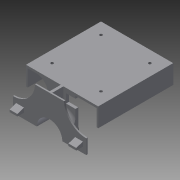
# Autodesk Inventor part: irkit-holder
Saved by Autodesk Inventor 2014 SP2 (Build 180247200, 247)
## iProperties
Created: 2017-11-24
Part Number: irkit-holder
Material: 一般
Document SubType Name: Modeling
Designer: hide
Density: 1 g/cm^3
Appearance: 既定
Author: hide
Autodesk Inventor part; units mm, degrees
ref_plane "YZ Plane" through (0, 0, 0) normal (1, 0, 0) x (0, 1, 0)
ref_plane "XZ Plane" through (0, 0, 0) normal (0, 1, 0) x (-1, 0, 0)
ref_plane "XY Plane" through (0, 0, 0) normal (0, 0, 1) x (1, 0, 0)
sketch "スケッチ1" plane through (0, 0, 0) normal (0, 1, 0) x (-1, 0, 0)
  arc A0 (11.5, 0) -> (-11.5, 0) centre (0, 0) ccw
  arc A1 (13, 0) -> (-13, 0) centre (0, 0) ccw
  line L0 (-13, 0) -> (-11.5, 0)
  line L1 (11.5, 0) -> (13, 0)
  dimension "d0" = 1.5
  dimension "d1" = 23
  constraints: 4 end point, 4 point on circle, 2 centre point, 2 coincident, 2 horizontal
  measures "d0" radial gap between concentric circles of A0 A1
  measures "d1" diameter of A0
extrude "押し出し1" add sketch "スケッチ1" along normal blind 12.5
sketch "スケッチ2" plane through (0, 12.5, 0) normal (0, 1, 0) x (1, 0, 0)
  arc A0 (-13, 0) -> (13, 0) centre (0, 0) ccw projected
  line L0 (13, 0) -> (11.5, 0) projected
  arc A1 (-11.5, 0) -> (11.5, 0) centre (0, 0) ccw projected
  line L1 (-11.5, 0) -> (-13, 0) projected
  line L2 (12, 0) -> (12, -30)
  line L3 (12, -30) -> (-13, -30)
  line L4 (-13, -30) -> (-13, 0)
  line L5 (-13, 0) -> (-11.5, 0)
  line L6 (11.5, 0) -> (12, 0)
  line L7 (12, -19.8001) -> (3.5501, -19.8001)
  line L8 (3.5501, -19.8001) -> (3.5501, -27.7778)
  line L9 (3.5501, -27.7778) -> (12, -27.7778)
  line L10 (12, -27.7778) -> (12, -19.8001)
  dimension "d4" = 30
  constraints: 18 end point, 5 parallel, 3 horizontal, 3 perpendicular, 2 point on circle, 1 point on line
  measures "d4" distance of L3.end L1.end
extrude "押し出し2" add sketch "スケッチ2" against normal blind 2.5 contours A0 L2 L7 L8 L9 L3 L4
sketch "スケッチ3" plane through (-13, 12.5, 30) normal (0, 0, 1) x (1, 0, 0)
  line L0 (0, 0) -> (25, 0) projected
  line L1 (25, -2.5) -> (0, -2.5) projected
  line L2 (-19.5, -2.5) -> (45.5, -2.5)
  line L3 (45.5, -2.5) -> (45.5, 65)
  line L4 (45.5, 65) -> (-19.5, 65)
  line L5 (-19.5, 65) -> (-19.5, -2.5)
  circle A0 centre (-9, 54.5) radius 1.25
  circle A1 centre (35, 54.5) radius 1.25
  circle A2 centre (-9, 10.5) radius 1.25
  circle A3 centre (35, 10.5) radius 1.25
  point P0 (13, -12.5)
  dimension "d7" = 65
  dimension "d8" = 0
  dimension "d9" = 65
  dimension "d10" = 32.5
  dimension "d13" = 2.5
  dimension "d14" = 2.5
  dimension "d15" = 2.5
  dimension "d16" = 2.5
  dimension "d17" = 44
  dimension "d18" = 44
  dimension "d19" = 0
  dimension "d20" = 0
  dimension "d21" = 10.5
  dimension "d22" = 10.5
  dimension "d23" = 44
  dimension "d24" = 0
  constraints: 8 end point, 4 centre point, 2 parallel, 1 horizontal, 1 perpendicular
  measures "d7" distance of L3.end L4.end
  measures "d8" distance between parallel lines of L1 L2
  measures "d9" distance between parallel lines of L0 L4
  measures "d10" distance from line of point (13, -12.5) L5
  measures "d13" diameter of A0
  measures "d14" diameter of A1
  measures "d15" diameter of A2
  measures "d16" diameter of A3
  measures "d17" distance of A1.centre A0.centre
  measures "d18" distance of A3.centre A1.centre
  measures "d19" vertical distance of A3.centre A2.centre
  measures "d20" vertical distance of A1.centre A0.centre
  measures "d21" distance from line of L4 A0.centre
  measures "d22" distance from line of L5 A0.centre
  measures "d23" distance of A2.centre A3.centre
  measures "d24" horizontal distance of A0.centre A2.centre
extrude "押し出し3" add sketch "スケッチ3" along normal blind 2
fillet "フィレット1" radius 10 1 edges at (-13, 11.25, 30)
sketch "スケッチ5" plane through (-13, 12.5, 30) normal (0, 0, -1) x (-1, 0, 0)
  line L0 (19.5, -2.5) -> (10, -2.5) projected
  line L1 (19.5, 65) -> (19.5, -2.5) projected
  line L2 (-25, -2.5) -> (-45.5, -2.5) projected
  line L3 (-45.5, 65) -> (-44, 65)
  line L4 (-44, 65) -> (-44, -2.5)
  line L5 (-44, -2.5) -> (-45.5, -2.5)
  line L6 (-45.5, -2.5) -> (-45.5, 65)
  line L7 (19.5, 65) -> (18, 65)
  line L8 (18, 65) -> (18, -2.5)
  line L9 (18, -2.5) -> (19.5, -2.5)
  line L10 (19.5, -2.5) -> (19.5, 65)
  point P0 (-13, -12.5)
  dimension "d26" = 1.5
  dimension "d27" = 1.5
  constraints: 16 end point, 4 parallel, 2 horizontal, 2 perpendicular, 2 point on line
  measures "d26" distance between parallel lines of L6 L4
  measures "d27" distance between parallel lines of L1 L8
extrude "押し出し4" add sketch "スケッチ5" along normal blind 15
sketch "スケッチ6" plane through (-13, 12.5, 30) normal (0, 0, -1) x (-1, 0, 0)
  circle A0 centre (-35, 10.5) radius 1.25 projected
  circle A1 centre (9, 10.5) radius 1.25 projected
  circle A2 centre (-35, 54.5) radius 1.25 projected
  circle A3 centre (9, 54.5) radius 1.25 projected
  circle A4 centre (-35, 54.5) radius 2.5
  circle A5 centre (-35, 10.5) radius 2.5
  circle A6 centre (9, 10.5) radius 2.5
  circle A7 centre (9, 54.5) radius 2.5
  point P0 (-13, -12.5)
  dimension "d30" = 5
  dimension "d31" = 5
  dimension "d32" = 5
  dimension "d33" = 5
  constraints: 4 centre point, 4 coincident
  measures "d30" diameter of A4
  measures "d31" diameter of A7
  measures "d32" diameter of A5
  measures "d33" diameter of A6
extrude "押し出し5" add sketch "スケッチ6" along normal blind 10
fillet "フィレット2" radius 5 1 edges at (-5.5, 12.5, 30)
sketch "スケッチ7" plane through (0, 0, 0) normal (0, -1, 0) x (1, 0, 0)
  arc A0 (11.5, 0) -> (-11.5, 0) centre (0, 0) ccw projected
  line L0 (13, 0) -> (13, 32)
  line L1 (13, 32) -> (-13, 32)
  line L2 (-13, 32) -> (-13, 0)
  line L3 (-13, 0) -> (-23, 0)
  line L4 (-23, 0) -> (-23, 10)
  line L5 (-23, 10) -> (-13, 10)
  line L6 (-13, 10) -> (-13, 0)
  line L7 (13, 0) -> (23, 0)
  line L8 (23, 0) -> (23, 10)
  line L9 (23, 10) -> (13, 10)
  line L10 (13, 10) -> (13, 0)
  line L11 (-13, 0) -> (-11.5, 0)
  line L12 (11.5, 0) -> (13, 0)
  line L13 (-23, 0) -> (-13, 0)
  line L14 (-13, 0) -> (-13, -10)
  line L15 (-13, -10) -> (-23, -10)
  line L16 (-23, -10) -> (-23, 0)
  line L17 (23, 0) -> (13, 0)
  line L18 (13, 0) -> (13, -10)
  line L19 (13, -10) -> (23, -10)
  line L20 (23, -10) -> (23, 0)
  line L21 (-13, 13) -> (-33, 13)
  line L22 (-33, 13) -> (-33, 0)
  line L23 (-33, 0) -> (-13, 0)
  line L24 (-13, 0) -> (-13, 13)
  line L25 (13, 0) -> (33, 0)
  line L26 (33, 0) -> (33, 13)
  line L27 (33, 13) -> (13, 13)
  line L28 (13, 13) -> (13, 0)
  dimension "d37" = 32
  dimension "d38" = 10
  dimension "d39" = 10
  dimension "d40" = 10
  dimension "d41" = 10
  dimension "d46" = 10
  dimension "d47" = 10
  dimension "d64" = 20
  dimension "d65" = 20
  dimension "d66" = 13
  dimension "d67" = 13
  dimension "d68" = 0
  constraints: 58 end point, 15 parallel, 8 horizontal, 8 perpendicular, 2 point on circle, 1 point on line
  measures "d37" distance of L1.end L2.end
  measures "d38" distance of L2.end L3.end
  measures "d39" distance of L0.start L7.end
  measures "d40" distance of L3.end L4.end
  measures "d41" distance of L7.end L8.end
  measures "d46" distance of L15.end L3.end
  measures "d47" distance of L19.end L7.end
  measures "d64" distance of L21.start L21.end
  measures "d65" distance of L26.end L27.end
  measures "d66" distance of L21.end L22.end
  measures "d67" distance of L25.end L26.end
  measures "d68" distance from line of A0.centre L23
extrude "押し出し6" add sketch "スケッチ7" along normal blind 1.3 contours A0 L11 L2 L1 L0 L12 | L0 L9 L8 L7 | L3 L4 L5 L2 | L0 L27 L26 L25 L8 L9 | L5 L4 L23 L22 L21 L2
fillet "フィレット4" radius 5 2 edges at (-2.5495, 10, 12.7475) (0, 0, 13)
sketch "スケッチ8" plane through (0, -1.3, 0) normal (0, -1, 0) x (1, 0, 0)
  line L0 (-13, -10) -> (-13, 0) projected
  line L1 (13, 0) -> (13, -10) projected
  line L2 (-30, 9) -> (-23, 9)
  line L3 (-23, 9) -> (-23, 5)
  line L4 (-23, 5) -> (-30, 5)
  line L5 (-30, 5) -> (-30, 9)
  line L6 (23, 9) -> (30, 9)
  line L7 (30, 9) -> (30, 5)
  line L8 (30, 5) -> (23, 5)
  line L9 (23, 5) -> (23, 9)
  line L10 (-33, 0) -> (-11.5, 0) projected
  line L11 (11.5, 0) -> (33, 0) projected
  dimension "d48" = 4
  dimension "d49" = 4
  dimension "d50" = 7
  dimension "d51" = 7
  dimension "d52" = 10
  dimension "d53" = 10
  dimension "d69" = 5
  dimension "d70" = 5
  constraints: 16 end point, 4 parallel, 2 horizontal, 2 perpendicular
  measures "d48" distance of L4.end L2.start
  measures "d49" distance of L8.end L6.start
  measures "d50" distance of L2.start L2.end
  measures "d51" distance of L6.start L6.end
  measures "d52" distance between parallel lines of L0 L3
  measures "d53" distance between parallel lines of L1 L9
  measures "d69" distance between parallel lines of L10 L4
  measures "d70" distance between parallel lines of L11 L8
extrude "押し出し7" add sketch "スケッチ8" along normal blind 6
chamfer "面取り1" distance 6 distance2 2 1 edges at (-26.5, -7.3, 9) measured on face at (-27.6667, -3.3, 9)
chamfer "面取り2" distance 6 distance2 2 1 edges at (26.5, -7.3, 9) measured on face at (25.3333, -3.3, 9)
fillet "フィレット5" radius 20 2 edges at (-13, -0.65, 13) (13, -0.65, 13)
sketch "スケッチ9" plane through (0, 0, 0) normal (1, 0, 0) x (0, 1, 0)
  arc A0 (-1.1136, 18.2387) -> (10.5299, 18.2387) centre (4.7082, 18.2387) ccw
  line L0 (10.5299, 18.2387) -> (10.8084, 18.2387)
  line L1 (10.8084, 18.2387) -> (10.8084, 32)
  line L2 (10.8084, 32) -> (-1.1136, 32)
  line L3 (-1.1136, 32) -> (-1.1136, 18.2387)
  line L4 (-1.3, 32) -> (-1.3, 13) projected
  line L5 (-1.3, 13) -> (0, 13) projected
  line L6 (0, 32) -> (0, 13) projected
  line L7 (0, 32) -> (-1.3, 32) projected
  point P0 (0, 0)
  dimension "d74" = 0
  constraints: 8 end point, 2 parallel, 2 point on circle, 1 centre point, 1 horizontal, 1 perpendicular
  measures "d74" distance between parallel lines of L2 L7
extrude "押し出し8" add sketch "スケッチ9" along normal mid plane 2.4 contours L3 L2 L6 A0 | L6 L2 L1 L0 A0
equation "\"d9\" = d7"
equation "\"d10\" = 0.5 * d7"
equation "\"d14\" = d13"
equation "\"d15\" = d13"
equation "\"d16\" = d13"
equation "\"d18\" = d17"
equation "\"d21\" = -0.5 * d17 + 0.5 * d7"
equation "\"d22\" = d21"
equation "\"d23\" = d17"
equation "\"d27\" = d26"
equation "\"d31\" = d30"
equation "\"d32\" = d30"
equation "\"d33\" = d30"
equation "\"d39\" = d38"
equation "\"d41\" = d40"
equation "\"d46\" = d40"
equation "\"d47\" = d40"
equation "\"d65\" = d64"
equation "\"d67\" = d66"
equation "\"d49\" = d48"
equation "\"d51\" = d50"
equation "\"d70\" = d69"
